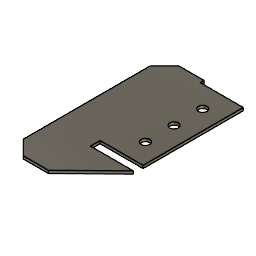
GPL H350 to 250G31_ (Autodesk Fusion 360 design; units mm, degrees)
Autodesk Fusion 360 part; units mm, degrees
sketch "スケッチ1" plane through (0, 0, 0) normal (0, 0, 1) x (1, 0, 0)
  line L0 (-3.5, 163) -> (-86.5, 163)
  line L1 (-86.5, 163) -> (-86.5, -163)
  line L2 (-86.5, -163) -> (-3.5, -163)
  line L3 (86.5, -55) -> (86.5, 155)
  line L4 (82.2546, 155) -> (-86.5, -163) construction
  line L5 (-3.5, 163) -> (-3.5, 155)
  line L6 (-3.5, 155) -> (86.5, 155)
  line L7 (-86.5, -163) -> (-3.5, -163) construction
  line L8 (86.5, -75) -> (-3.5, -163)
  line L9 (86.5, -75) -> (-3.5, -75)
  line L10 (-3.5, -75) -> (-3.5, -55)
  line L11 (-3.5, -55) -> (86.5, -55)
  line L12 (-86.5, 163) -> (29.1871, -55) construction
  line L13 (39.8006, -75) -> (55.7541, -105.0627) construction
  dimension "d2" = 326
  dimension "d5" = 83
  dimension "d7" = 90
  dimension "d8" = 20
  constraint horizontal L0
  constraint perpendicular L0 L1
  constraint parallel L0 L2
  constraint parallel L1 L3
  constraint coincident L4 origin
  constraint coincident origin L12
  constraint vertical L5
  constraint horizontal L6
  constraint coincident L6 L4.start
  constraint perpendicular L1 L7
  constraint coincident L8 L13.end
  constraint horizontal L9
  constraint vertical L10
  constraint horizontal L11
  constraint coincident L11 L12.end
  constraint coincident L9 L13.start
  constraint collinear L12 L13
  measures "d2" distance of L0.end L1.end
  measures "d5" distance of L1.end L2.end
  measures "d7" distance of L8.start L9.end
  measures "d8" distance of L8.start L3.start
extrude "押し出し1" add sketch "スケッチ1" along normal blind 6
chamfer "面取り1" distance 30 angle 45 2 edges at (-86.5, -163, 3) (-86.5, 163, 3)
sketch "スケッチ2" plane through (0, 0, 6) normal (0, 0, 1) x (-1, 0, 0)
  line L0 (56.5, -163) -> (86.5, -133)
  line L1 (86.5, -133) -> (86.5, 133)
  line L2 (86.5, 133) -> (56.5, 163)
  line L3 (56.5, 163) -> (3.5, 163)
  line L4 (3.5, 163) -> (-86.5, 75)
  line L5 (-86.5, 75) -> (3.5, 75)
  line L6 (3.5, 75) -> (3.5, 55)
  line L7 (3.5, 55) -> (-86.5, 55)
  line L8 (-86.5, 55) -> (-86.5, -155)
  line L9 (-86.5, -155) -> (3.5, -155)
  line L10 (3.5, -155) -> (3.5, -163)
  line L11 (3.5, -163) -> (56.5, -163)
  line L12 (-86.5, -155) -> (-46.5, -155) construction
  line L13 (-46.5, -155) -> (-46.5, -110) construction
  line L14 (-46.5, -110) -> (-86.5, -110) construction
  line L15 (-86.5, -110) -> (-86.5, -155) construction
  line L16 (-46.5, -110) -> (-46.5, -50) construction
  line L17 (-46.5, -50) -> (-46.5, 10) construction
  point P0 (-46.5, -110)
  point P1 (-46.5, -50)
  dimension "d12" = 40
  dimension "d13" = 45
  dimension "d14" = 60
  dimension "d15" = 60
  constraint horizontal L12
  constraint vertical L13
  constraint horizontal L14
  constraint vertical L15
  constraint coincident L8.end L9.start
  constraint perpendicular L14 L16
  constraint parallel L16 L17
  constraint coincident P0 L13.end
  constraint coincident P1 L16.end
  measures "d12" distance of L8.end L12.end
  measures "d13" distance of L8.end L14.end
  measures "d14" distance of P0 P1
  measures "d15" distance of P1 L17.end
hole "穴1" at (46.5, 110, 6) at (46.5, 50, 6) at (46.5, -10, 6) direction (0, 0, -1) diameter 18 end through all
equation "d5 = 30 mm + 53 mm"
